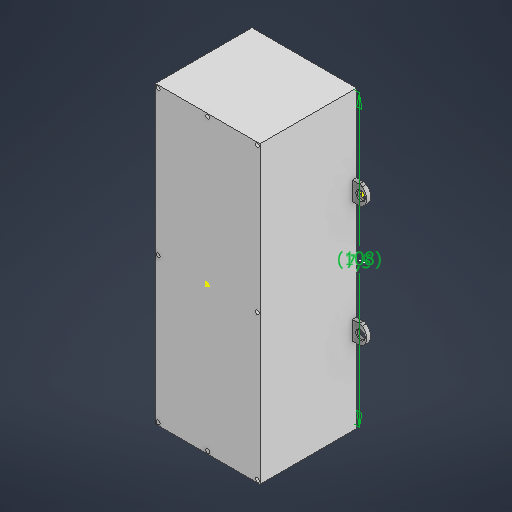
# Autodesk Inventor part: batterycase
Saved by Autodesk Inventor 2026.1 (Build 301233000, 233)
## iProperties
Created: 2026-05-03
Part Number: batterycase
Material: Generic
Document SubType Name: Modeling
Designer: ayjuni03
Density: 1 g/cm^3
Appearance: Default
Mass: 23.788 g
Surface Area: 304.974 cm^2
Volume: 23.788 cm^3
Author: ayjuni03
Autodesk Inventor part; units mm, degrees
ref_plane "YZ Plane" through (0, 0, 0) normal (1, 0, 0) x (0, 1, 0)
ref_plane "XZ Plane" through (0, 0, 0) normal (0, 1, 0) x (-1, 0, 0)
ref_plane "XY Plane" through (0, 0, 0) normal (0, 0, 1) x (1, 0, 0)
sketch "Sketch1" plane through (0, 0, 0) normal (0, 0, 1) x (1, 0, 0)
  line L0 (0, 0) -> (-16.5, 0) construction
  line L1 (-16.5, 0) -> (16.5, 0) construction
  line L2 (-16.5, 0) -> (-16.5, 52)
  line L3 (-16.5, 52) -> (-16.5, -52)
  line L4 (16.5, 0) -> (16.5, 52)
  line L5 (16.5, 52) -> (16.5, -52)
  line L6 (-16.5, 52) -> (16.5, 52)
  line L7 (-16.5, -52) -> (16.5, -52)
  dimension "d0" = 16.5
  dimension "d1" = 33
  dimension "d2" = 52
  dimension "d3" = 104
  dimension "d4" = 52
  dimension "d5" = 104
  constraints: 16 end point, 3 point on line, 2 vertical, 1 horizontal
  measures "d0" distance of L0.start L0.end
  measures "d1" distance of L0.end L1.end
  measures "d2" distance of L0.end L2.end
  measures "d3" distance of L2.end L3.end
  measures "d4" distance of L1.end L4.end
  measures "d5" distance of L4.end L5.end
extrude "Extrusion1" add sketch "Sketch1" along normal blind 1
sketch "Sketch2" plane through (0, 0, 1) normal (0, 0, 1) x (1, 0, 0)
  line L0 (16.5, 52) -> (-16.5, 52) projected
  line L1 (16.5, 52) -> (-16.5, 52)
  line L2 (16.5, -52) -> (16.5, 52) projected
  line L3 (16.5, 52) -> (16.5, -52)
  line L4 (-16.5, 52) -> (-16.5, -52) construction
  line L5 (-16.5, 0) -> (-24, 0) construction
  line L6 (16.5, 0) -> (24, 0) construction
  line L7 (-16.5, 52) -> (-18.5, 52)
  line L8 (-18.5, 52) -> (-18.5, 54)
  line L9 (-18.5, 54) -> (18.5, 54)
  line L10 (18.5, 54) -> (18.5, 52)
  line L11 (18.5, 52) -> (16.5, 52)
  line L12 (-16.5, 52) -> (-16.5, -52)
  line L13 (-18.5, 52) -> (-18.5, -54)
  line L14 (-18.5, -54) -> (-16.5, -54)
  line L15 (-16.5, -52) -> (16.5, -52) projected
  line L16 (-16.5, -52) -> (16.5, -52)
  line L17 (16.5, -52) -> (16.5, -54)
  line L18 (16.5, -54) -> (-16.5, -54)
  line L19 (-16.5, -54) -> (-16.5, -52)
  line L20 (16.5, -54) -> (18.5, -54)
  line L21 (18.5, -54) -> (18.5, 52)
  point P0 (0, 0)
  dimension "d8" = 7.5
  dimension "d9" = 7.5
  dimension "d10" = 2
  dimension "d11" = 2
  dimension "d12" = 37
  dimension "d13" = 106
  constraints: 36 end point, 8 perpendicular, 4 collinear, 4 point on line, 2 horizontal, 2 midpoint, 1 parallel, 1 vertical
  measures "d8" distance of L5.start L5.end
  measures "d9" distance of L6.start L6.end
  measures "d10" distance of L0.end L7.end
  measures "d11" distance of L7.end L8.end
  measures "d12" distance of L8.end L9.end
  measures "d13" distance of L7.end L13.end
extrude "Extrusion2" add sketch "Sketch2" against normal blind 36 contours L11 L21 L20 L17 L2 | L0 L7 L8 L9 L10 L11 | L12 L19 L14 L13 L7 | L17 L18 L19 L15
sketch "Sketch3" plane through (0, 0, -35) normal (0, 0, -1) x (-1, 0, 0)
  line L0 (-18.5, -54) -> (18.5, -54) projected
  line L1 (-18.5, 54) -> (-18.5, -54) projected
  line L2 (-18.5, -54) -> (-18.5, 54)
  line L3 (-16.5, -52) -> (-16.5, 52) construction
  line L4 (-16.5, 0) -> (-24, 0) construction
  point P0 (0, 0)
  dimension "d16" = 108
  dimension "d17" = 7.5
  constraints: 4 end point, 1 collinear, 1 horizontal, 1 midpoint
  measures "d16" distance of L0.start L1.start
  measures "d17" distance of L4.start L4.end
sketch "Sketch4" plane through (-18.5, -54, 1) normal (0, -1, 0) x (1, 0, 0)
  line L0 (37, 0) -> (37, -36) projected
  line L1 (37, -36) -> (37, 0)
  line L2 (0, 0) -> (37, 0) projected
  line L3 (37, 0) -> (36, 0)
  line L4 (36, 0) -> (30, 0)
  line L5 (30, 0) -> (30, -36)
  line L6 (37, -36) -> (0, -36) projected
  line L7 (36, 0) -> (36, -36)
  line L8 (35, -1) -> (35, -36) projected
  line L9 (30, -36) -> (36, -36)
  line L10 (30, -36) -> (30, -31)
  line L11 (30, -31) -> (36, -31)
  line L12 (30, 0) -> (30, -5)
  line L13 (30, -5) -> (36, -5)
  line L14 (30, -5) -> (29, -5)
  line L15 (35, -1) -> (2, -1) projected
  line L16 (29, -5) -> (27.5, -5)
  line L17 (27.5, -5) -> (27.5, -31)
  line L18 (27.5, -31) -> (30, -31)
  point P0 (18.5, -1)
  dimension "d18" = 1
  dimension "d19" = 6
  dimension "d20" = 5
  dimension "d21" = 5
  dimension "d22" = 1
  dimension "d23" = 1.5
  constraints: 28 end point, 8 point on line, 6 perpendicular, 2 parallel, 1 collinear
  measures "d18" distance of L0.start L3.end
  measures "d19" distance of L3.end L4.end
  measures "d20" distance of L5.end L10.end
  measures "d21" distance of L4.end L12.end
  measures "d22" distance of L12.end L14.end
  measures "d23" distance of L14.end L16.end
extrude "Extrusion3" cut sketch "Sketch4" against normal blind 36 contours L7 L11 L8 L13 | L8 L11 L5 L13 | L5 L18 L17 L16 L14
sketch "Sketch5" plane through (0, 0, 1) normal (0, 0, 1) x (1, 0, 0)
  point P0 (0, 0)
sketch "Sketch6" plane through (-18.5, 54, 1) normal (0, 1, 0) x (1, 0, 0)
  line L0 (37, 0) -> (37, 36)
  line L1 (0, 0) -> (0, 36) projected
  line L2 (37, 36) -> (0, 36)
  line L3 (0, 36) -> (0, 0)
  line L4 (0, 0) -> (37, 0)
  point P0 (18.5, 1)
  constraints: 8 end point, 3 perpendicular
extrude "Extrusion4" add sketch "Sketch6" along normal blind 1
sketch "Sketch7" plane through (18.5, -54, 1) normal (1, 0, 0) x (0, 0, -1)
  line L0 (36, 109) -> (0, 109) projected
  line L1 (0, 109) -> (36, 109)
  line L2 (1, 106) -> (36, 106) projected
  line L3 (36, 109) -> (36, 0)
  line L4 (36, 0) -> (0, 0)
  line L5 (0, 0) -> (0, 109)
  point P0 (1, 54)
  constraints: 8 end point, 3 perpendicular, 1 parallel
extrude "Extrusion5" add sketch "Sketch7" along normal blind 1
sketch "Sketch8" plane through (-18.5, -54, -35) normal (-1, 0, 0) x (0, 0, 1)
  line L0 (0, 0) -> (0, 109) projected
  line L1 (36, 109) -> (36, 0) projected
  line L2 (0, 109) -> (36, 109)
  line L3 (36, 109) -> (36, 0)
  line L4 (36, 0) -> (0, 0)
  line L5 (0, 0) -> (0, 109)
  point P0 (35, 54)
  constraints: 8 end point, 3 perpendicular, 1 horizontal
extrude "Extrusion6" add sketch "Sketch8" along normal blind 1
sketch "Sketch9" plane through (19.5, -54, -35) normal (0, -1, 0) x (1, 0, 0)
  line L0 (0, 0) -> (0, 36) projected
  line L1 (-39, 36) -> (-39, 0) projected
  line L2 (0, 0) -> (-39, 0)
  line L3 (-39, 0) -> (-39, 36)
  line L4 (-39, 36) -> (0, 36)
  line L5 (0, 36) -> (0, 0)
  line L6 (-2, 5) -> (-10.5, 5) projected
  line L7 (-2, 5) -> (-10.5, 5)
  line L8 (-10.5, 5) -> (-10.5, 31) projected
  line L9 (-10.5, 5) -> (-10.5, 31)
  line L10 (-10.5, 31) -> (-2, 31)
  line L11 (-2, 31) -> (-2, 5)
  point P0 (-19.5, 35)
  constraints: 16 end point, 6 perpendicular, 2 horizontal
extrude "Extrusion7" add sketch "Sketch9" along normal blind 1
sketch "Sketch10" plane through (0, 0, -35) normal (0, 0, -1) x (-1, 0, 0)
  line L0 (-16.5, -52) -> (-16.5, 52) construction
  line L1 (-16.5, 0) -> (-17.5, 0) construction
  line L2 (-17.5, 0) -> (-17.5, 52)
  line L3 (-16.5, 52) -> (16.5, 52) projected
  line L4 (-17.5, 52) -> (-16.5, 52)
  line L5 (-16.5, 52) -> (-16.5, 53)
  line L6 (-16.5, 53) -> (-17.5, 53)
  line L7 (-17.5, 52) -> (-17.5, 53)
  line L8 (-16.5, 53) -> (17.5, 53)
  line L9 (17.5, 53) -> (17.5, 52)
  line L10 (17.5, 52) -> (16.5, 52)
  line L11 (17.5, 52) -> (17.5, -53)
  line L12 (17.5, -53) -> (16.5, -53)
  line L13 (16.5, 52) -> (16.5, -52) projected
  line L14 (16.5, -52) -> (16.5, -53)
  line L15 (16.5, -53) -> (-17.5, -53)
  line L16 (-17.5, -53) -> (-17.5, -52)
  line L17 (16.5, -52) -> (-16.5, -52) projected
  line L18 (-17.5, -52) -> (-16.5, -52)
  line L19 (-17.5, -52) -> (-17.5, 0)
  line L20 (-16.5, -52) -> (-16.5, -18) projected
  line L21 (-16.5, -52) -> (16.5, -52)
  line L22 (16.5, 52) -> (16.5, -52) projected
  line L23 (16.5, 52) -> (16.5, -52)
  line L24 (-16.5, 52) -> (-16.5, -52)
  line L25 (-16.5, 52) -> (16.5, 52)
  point P0 (0, 0)
  dimension "d34" = 1
  dimension "d35" = 1
  dimension "d36" = 34
  dimension "d37" = 105
  dimension "d38" = 34
  dimension "d39" = 104
  constraints: 40 end point, 9 perpendicular, 4 point on line, 3 collinear, 2 horizontal, 2 vertical, 1 midpoint, 1 parallel
  measures "d34" distance of L1.start L1.end
  measures "d35" distance of L0.end L5.end
  measures "d36" distance of L5.end L8.end
  measures "d37" distance of L9.end L11.end
  measures "d38" distance of L12.end L15.end
  measures "d39" distance of L0.end L0.start
extrude "Extrusion8" cut sketch "Sketch10" against normal blind 35 contours L2 L4 L24 L20 L18 L19 | L7 L6 L5 L4 | L18 L17 L14 L15 L16 | L5 L8 L9 L10 L3 | L10 L11 L12 L14 L13
sketch "Sketch11" plane through (0, 0, -35) normal (0, 0, -1) x (-1, 0, 0)
  line L0 (-19.5, 55) -> (-19.5, -55) construction
  line L1 (-19.5, 0) -> (-21, 0) construction
  line L2 (19.5, 55) -> (19.5, -55) construction
  line L3 (19.5, 0) -> (21, 0) construction
  line L4 (19.5, 55) -> (19.5, 24) construction
  line L5 (19.5, 55) -> (19.5, -21) construction
  line L6 (19.5, 24) -> (19.5, 21) construction
  line L7 (19.5, 22.5) -> (22.5, 22.5) construction
  circle A0 centre (22.5, 22.5) radius 1.5
  line L8 (19.5, -21) -> (19.5, -24) construction
  line L9 (19.5, -22.5) -> (22.5, -22.5) construction
  circle A1 centre (22.5, -22.5) radius 1.5
  line L10 (-19.5, 55) -> (-19.5, 24) construction
  line L11 (-19.5, 24) -> (-19.5, 21) construction
  line L12 (-19.5, 22.5) -> (-22.5, 22.5) construction
  circle A2 centre (-22.5, 22.5) radius 1.5
  line L13 (-19.5, 55) -> (-19.5, -21) construction
  line L14 (-19.5, -21) -> (-19.5, -24) construction
  line L15 (-19.5, -22.5) -> (-22.5, -22.5) construction
  circle A3 centre (-22.5, -22.5) radius 1.5
  line L16 (22.5016, 21) -> (22.5016, 19) construction
  line L17 (22.4741, 23.9998) -> (22.4741, 25.9998) construction
  arc A4 (23.1357, 19.3529) -> (23.0988, 25.66) centre (20.9722, 22.4939) ccw
  line L18 (19.5, 25.9998) -> (21.9836, 25.9998)
  line L19 (22.0012, 19) -> (19.5, 19)
  arc A5 (23.0988, 25.66) -> (21.9836, 25.9998) centre (21.9836, 23.9998) ccw
  arc A6 (22.0012, 19) -> (23.1357, 19.3529) centre (22.0012, 21) ccw
  line L20 (19.5, 25.9998) -> (19.5, 19)
  line L21 (22.5, -22.5) -> (22.5, -21) construction
  line L22 (22.5, -21) -> (22.5, -19) construction
  line L23 (22.5, -19) -> (22.5, -26) construction
  arc A7 (23.1294, -25.6536) -> (23.1294, -19.3464) centre (20.9841, -22.5) ccw
  line L24 (22.0045, -19) -> (19.5, -19)
  line L25 (22.0045, -26) -> (19.5, -26)
  line L26 (19.5, 55) -> (19.5, -55) projected
  line L27 (19.5, -19) -> (19.5, -26)
  arc A8 (23.1294, -19.3464) -> (22.0045, -19) centre (22.0045, -21) ccw
  arc A9 (22.0045, -26) -> (23.1294, -25.6536) centre (22.0045, -24) ccw
  line L28 (-22.5, -22.5) -> (-22.5, -19) construction
  line L29 (-22.5, -19) -> (-22.5, -26) construction
  arc A10 (-23.1293, -19.3462) -> (-23.1293, -25.6538) centre (-20.9845, -22.5) ccw
  line L30 (-22.0046, -19) -> (-19.5, -19)
  line L31 (-22.0046, -26) -> (-19.5, -26)
  arc A11 (-22.0046, -19) -> (-23.1293, -19.3462) centre (-22.0046, -21) ccw
  arc A12 (-23.1293, -25.6538) -> (-22.0046, -26) centre (-22.0046, -24) ccw
  line L32 (-22.5, 22.5) -> (-22.5, 26) construction
  line L33 (-22.5, 26) -> (-22.5, 19) construction
  arc A13 (-23.1226, 25.6584) -> (-23.1293, 19.3462) centre (-20.9845, 22.5) ccw
  line L34 (-22.0102, 26.0022) -> (-19.5, 26.0132)
  line L35 (-22.0046, 19) -> (-19.5, 19)
  line L36 (-19.5, 26.0132) -> (-19.5, 19)
  arc A14 (-22.0102, 26.0022) -> (-23.1226, 25.6584) centre (-22.0014, 24.0022) ccw
  arc A15 (-23.1293, 19.3462) -> (-22.0046, 19) centre (-22.0046, 21) ccw
  line L37 (-19.5, -19) -> (-19.5, -26)
  point P0 (0, 0)
  dimension "d49" = 3
  dimension "d42" = 1.5
  dimension "d43" = 1.5
  dimension "d44" = 31
  dimension "d45" = 76
  dimension "d46" = 3
  dimension "d47" = 3
  dimension "d48" = 3
  dimension "d50" = 31
  dimension "d51" = 3
  dimension "d52" = 3
  dimension "d53" = 76
  dimension "d54" = 3
  dimension "d55" = 3
  dimension "d56" = 2
  dimension "d57" = 2
  dimension "d58" = 2
  dimension "d59" = 2
  dimension "d60" = 2
  dimension "d61" = 7
  dimension "d62" = 3.8142
  dimension "d63" = 3.814
  dimension "d64" = 2
  dimension "d65" = 3.5
  dimension "d66" = 7
  dimension "d67" = 3.814
  dimension "d68" = 2
  dimension "d69" = 3.5
  dimension "d70" = 7
  dimension "d71" = 3.814
  dimension "d72" = 2
  constraints: 70 end point, 35 point on circle, 27 point on line, 16 tangent, 15 centre point, 6 horizontal, 6 midpoint, 6 perpendicular, 6 vertical, 4 coincident, 3 collinear, 3 equal radius, 1 parallel, 1 vertical alignment, 4 other
  measures "d42" distance of L1.start L1.end
  measures "d43" distance of L3.start L3.end
  measures "d44" distance of L2.start L4.end
  measures "d45" distance of L2.start L5.end
  measures "d46" distance of L4.end L6.end
  measures "d47" distance of L7.start L7.end
  measures "d48" distance of L5.end L8.end
  measures "d50" distance of L0.start L10.end
  measures "d51" distance of L12.start L12.end
  measures "d52" diameter of A2
  measures "d53" distance of L0.start L13.end
  measures "d54" distance of L13.end L14.end
  measures "d55" diameter of A3
  measures "d56" distance of L16.start L16.end
  measures "d57" distance of L17.start L17.end
  measures "d58" radius of A5
  measures "d59" radius of A6
  measures "d60" distance of L21.end L22.end
  measures "d61" distance of L22.end L23.end
  measures "d62" radius of A7
  measures "d63" radius of A4
  measures "d64" radius of A8
  measures "d65" distance of L28.start L28.end
  measures "d66" distance of L28.end L29.end
  measures "d67" radius of A10
  measures "d68" radius of A11
  measures "d69" distance of L32.start L32.end
  measures "d70" distance of L32.end L33.end
  measures "d71" radius of A13
  measures "d72" radius of A14
extrude "Extrusion9" add sketch "Sketch11" against normal blind 1.5
sketch "Sketch12" plane through (0, 0, -35) normal (0, 0, -1) x (-1, 0, 0)
  circle A0 centre (-22.5, 22.5) radius 1.5 construction
  line L0 (-22.5, 24) -> (-22.5, 21) construction
  circle A1 centre (-22.5, 22.5) radius 1.5
  circle A2 centre (-22.5, -22.5) radius 1.5 construction
  line L1 (-22.5, -22.5) -> (-22.5, -21) construction
  line L2 (-22.5, -22.5) -> (-22.5, -24) construction
  circle A3 centre (-22.5, -22.5) radius 1.5 projected
  circle A4 centre (-22.5, -22.5) radius 1.5
  circle A5 centre (22.5, -22.5) radius 1.5 construction
  line L3 (22.5, -22.5) -> (22.5, -21) construction
  line L4 (22.5, -22.5) -> (22.5, -24) construction
  circle A6 centre (22.5, -22.5) radius 1.5
  circle A7 centre (22.5, 22.5) radius 1.5 construction
  line L5 (22.5, 22.5) -> (22.5, 24) construction
  line L6 (22.5, 22.5) -> (22.5, 21) construction
  circle A8 centre (22.5, 22.5) radius 1.5
  point P0 (0, 0)
  constraints: 14 end point, 8 point on circle, 4 centre point, 4 coincident, 4 vertical, 3 concentric, 3 point on line
sketch "Sketch13" plane through (0, 0, -35) normal (0, 0, -1) x (-1, 0, 0)
  point P0 (0, 0)
chamfer "Chamfer1" distance 0.3083 angle 45 2 edges at (-21, 22.5, -35) (-21, 22.5, -33.5)
chamfer "Chamfer2" distance 0.3083 angle 45 2 edges at (24, 22.5, -35) (24, 22.5, -33.5)
chamfer "Chamfer3" distance 0.3083 angle 45 2 edges at (24, -22.5, -33.5) (24, -22.5, -35)
chamfer "Chamfer4" distance 0.3083 angle 45 2 edges at (-21, -22.5, -33.5) (-21, -22.5, -35)
sketch "Sketch14" plane through (0, 0, -35) normal (0, 0, -1) x (-1, 0, 0)
  point P0 (0, 0)
sketch "Sketch15" plane through (0, 0, 0) normal (0, 1, 0) x (-1, 0, 0)
  point P0 (0, 0)
sketch "Sketch16" plane through (0, 0, -35) normal (0, 0, -1) x (-1, 0, 0)
  line L0 (-17.5, -53) -> (-17.5, 53) construction
  line L1 (-17.5, 53) -> (-18.4998, 53.9998) construction
  circle A0 centre (-18.4998, 53.9998) radius 0.75
  line L2 (17.5, 53) -> (17.5, -53) construction
  line L3 (17.5, 53) -> (18.4998, 53.9998) construction
  circle A1 centre (18.4998, 53.9998) radius 0.75
  line L4 (17.5, -53) -> (-17.5, -53) construction
  line L5 (-17.5, -53) -> (-18.4998, -53.9998) construction
  circle A2 centre (-18.4998, -53.9998) radius 0.75
  line L6 (17.5, -53) -> (18.4998, -53.9998) construction
  circle A3 centre (18.4998, -53.9998) radius 0.75
  line L7 (18.4998, 53.2498) -> (18.4998, -53.2498) construction
  line L8 (19.5, -26) -> (19.5, -55) construction
  line L9 (-18.4998, -53.2498) -> (-18.4786, 53.2501) construction
  line L10 (-18.4786, 53.2501) -> (-18.4892, 0.0001) construction
  circle A4 centre (-18.4892, 0.0001) radius 0.75
  circle A5 centre (18.4998, 0) radius 0.75
  point P0 (0, 0)
  dimension "d88" = 1.5
  dimension "d90" = 1.5
  dimension "d92" = 1.5
  dimension "d94" = 1.5
  dimension "d87" = 1.414
  dimension "d89" = 1.414
  dimension "d91" = 1.414
  dimension "d93" = 1.414
  dimension "d95" = 106.5
  dimension "d96" = 53.25
  dimension "d97" = 1.5
  dimension "d98" = 1.5
  constraints: 14 end point, 5 coincident, 3 vertical alignment, 2 centre point, 2 midpoint, 1 parallel, 9 other
  measures "d87" distance of L0.end L1.end
  measures "d89" distance of L2.start L3.end
  measures "d91" distance of L0.start L5.end
  measures "d93" distance of L2.end L6.end
  measures "d95" distance of L9.start L9.end
  measures "d96" distance of L9.end L10.end
  measures "d97" diameter of A4
  measures "d98" diameter of A5
extrude "Extrusion10" cut sketch "Sketch16" against normal blind 40
sketch "Sketch17" plane through (0, 0, -35) normal (0, 0, -1) x (-1, 0, 0)
  circle A0 centre (-18.4998, -53.9998) radius 0.75 construction
  line L0 (-18.4998, -53.9998) -> (18.5002, -53.9998) construction
  line L1 (18.5002, -53.9998) -> (0.0002, -53.9998) construction
  circle A1 centre (0.0002, -53.9998) radius 0.75
  line L2 (-18.4998, -53.9998) -> (-18.4998, 0) construction
  point P0 (0, 0)
  dimension "d101" = 37
  dimension "d102" = 18.5
  dimension "d103" = 1.5
  constraints: 6 end point, 1 centre point, 1 coincident, 1 horizontal, 1 midpoint, 1 vertical
  measures "d101" distance of L0.start L0.end
  measures "d102" distance of L0.end L1.end
  measures "d103" diameter of A1
extrude "Extrusion11" cut sketch "Sketch17" against normal blind 40
sketch "Sketch18" plane through (0, 0, -35) normal (0, 0, -1) x (-1, 0, 0)
  circle A0 centre (-18.4998, 53.9998) radius 0.75 construction
  line L0 (-18.4998, 53.9998) -> (0, 53.9998) construction
  circle A1 centre (0, 53.9998) radius 0.75
  point P0 (0, 0)
  dimension "d106" = 1.5
  constraints: 2 end point, 1 centre point, 1 coincident, 1 horizontal
  measures "d106" diameter of A1
extrude "Extrusion12" cut sketch "Sketch18" against normal blind 40
sketch "Sketch19" plane through (0, 0, -35) normal (0, 0, -1) x (-1, 0, 0)
  circle A0 centre (-22.5, 22.5) radius 1.8083 construction
  line L0 (-20.6917, 22.5) -> (-17.5, 22.5) construction
  line L1 (-17.5, -53) -> (-17.5, 53) construction
  line L2 (-20.6917, 22.5) -> (-19.0959, 22.5) construction
  point P0 (0, 0)
  constraints: 4 end point, 1 horizontal, 1 horizontal alignment, 1 midpoint, 1 point on line, 1 other
sketch "Sketch20" plane through (0, 0, 0) normal (0, 0, -1) x (-1, 0, 0)
  line L0 (-17.5, 53) -> (17.5, 53) construction
  line L1 (-17.5, -53) -> (-17.5, 53) construction
  line L2 (-17.5, 53) -> (-17.5, -53) construction
  line L3 (17.5, 53) -> (17.5, -53) construction
  line L4 (-17.5, -53) -> (17.5, -53) construction
  line L5 (17.5, -53) -> (17.5, 53) construction
  line L6 (17.5, 53) -> (-17.5, 53) construction
  point P0 (0, 0)
  constraints: 8 end point, 2 perpendicular, 1 collinear, 1 vertical
thread "Thread1" size "M3x0.5" class "6H" standard "ISO Metric profile" full length
thread "Thread2" size "M3x0.5" class "6H" standard "ISO Metric profile" full length
thread "Thread3" size "M3x0.5" class "6H" standard "ISO Metric profile" full length
thread "Thread4" size "M3x0.5" class "6H" standard "ISO Metric profile" full length
body "Solid1"
